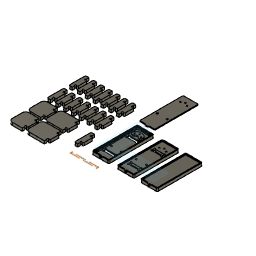
Basic Wood Geta with cavity v43 (Autodesk Fusion 360 design; units mm, degrees)
Autodesk Fusion 360 part; units mm, degrees
sketch "GetaDown" plane through (0, 0, 0) normal (0, 0, 1) x (1, 0, 0)
  line L0 (0, 0) -> (270, 0)
  line L1 (270, 0) -> (270, 100)
  line L2 (270, 100) -> (0, 100)
  line L3 (0, 100) -> (0, 0)
  line L4 (10, 90) -> (10, 10)
  line L5 (10, 10) -> (260, 10)
  line L6 (260, 10) -> (260, 90)
  line L7 (260, 90) -> (10, 90)
  dimension "d71" = 270
  dimension "d72" = 100
  constraint horizontal L0
  constraint vertical L1
  constraint horizontal L2
  constraint vertical L3
  constraint coincident L0.start L3.end
  measures "d71" distance of L0.start L0.end
  measures "d72" distance of L0.start L2.end
extrude "Extrude5" add sketch "GetaDown" along normal blind 5.6 contours L4 L5 L6 L7 makes body 1
extrude "Extrude12" add sketch "GetaDown" along normal blind 17.1 bodies 1
fillet "Fillet3" radius 6 4 edges at (0, 100, 8.55) (0, 0, 8.55) (270, 100, 8.55) (270, 0, 8.55) on bodies 1
fillet "Fillet7" radius 6 4 edges at (260, 90, 11.35) (260, 10, 11.35) (10, 90, 11.35) (10, 10, 11.35) on bodies 1
sketch "GetaUp" plane through (0, 0, 5.6) normal (0, 0, 1) x (-1, 0, 0)
  line L0 (0, 0) -> (-270, 0)
  line L1 (-270, 0) -> (-270, -100)
  line L2 (-270, -100) -> (0, -100)
  line L3 (0, -100) -> (0, 0)
  line L4 (-254, -90) -> (-16, -90)
  line L5 (-10, -84) -> (-10, -16)
  line L6 (-16, -10) -> (-254, -10)
  line L7 (-260, -16) -> (-260, -84)
  arc A0 (-10, -16) -> (-16, -10) centre (-16, -16) ccw
  arc A1 (-254, -10) -> (-260, -16) centre (-254, -16) ccw
  arc A2 (-260, -84) -> (-254, -90) centre (-254, -84) ccw
  arc A3 (-16, -90) -> (-10, -84) centre (-16, -84) ccw
  point P0 (-135, -90)
  point P1 (-135, -10)
  dimension "d17" = 270
  dimension "d18" = 100
  constraint horizontal L0
  constraint vertical L1
  constraint horizontal L2
  constraint vertical L3
  constraint midpoint L4 P0
  constraint midpoint L6 P1
  measures "d17" distance of L0.start L0.end
  measures "d18" distance of L0.start L2.end
extrude "Extrude7" add sketch "GetaUp" along normal blind 5 separate body contours L0 L1 L2 L3 | L4 L5 L6 L7 A0 A1 A2 A3 makes body 2
move_body "Move10" bodies 2 to x (1, 0, 0) y (0, 1, 0) z (0, 0, 1) at (0, 0, 17.1)
sketch "GetaBothPartHoles" plane through (0, 0, 5.6) normal (0, 0, 1) x (-1, 0, 0)
  circle A0 centre (-94.8, -80) radius 5
  circle A1 centre (-94.8, -20) radius 5
  circle A2 centre (-233.4, -50) radius 4
  circle A3 centre (-223.4, -70) radius 4
  circle A4 centre (-223.4, -30) radius 4
  line L0 (-254, -90) -> (-16, -90)
  line L1 (-10, -84) -> (-10, -16)
  line L2 (-16, -10) -> (-254, -10)
  line L3 (-260, -16) -> (-260, -84)
  arc A5 (-10, -16) -> (-16, -10) centre (-16, -16) ccw
  arc A6 (-254, -10) -> (-260, -16) centre (-254, -16) ccw
  arc A7 (-260, -84) -> (-254, -90) centre (-254, -84) ccw
  arc A8 (-16, -90) -> (-10, -84) centre (-16, -84) ccw
  line L4 (-10, -50) -> (-223.4, -50) construction
  line L5 (-223.4, -50) -> (-223.4, -70) construction
  line L6 (-223.4, -50) -> (-233.4, -50) construction
  line L7 (-223.4, -50) -> (-223.4, -30) construction
  dimension "d26" = 10
  dimension "d27" = 10
  dimension "d28" = 8
  dimension "d66" = 8
  dimension "d67" = 8
  dimension "d191" = 213.4
  dimension "d193" = 20
  dimension "d194" = 10
  dimension "d195" = 20
  constraint midpoint L1 L4.start
  constraint perpendicular L1 L4
  constraint vertical L5
  constraint horizontal L6
  constraint perpendicular L4 L7
  constraint coincident A2.centre L6.end
  constraint coincident A3.centre L5.end
  constraint coincident A4.centre L7.end
  measures "d26" diameter of A0
  measures "d27" diameter of A1
  measures "d28" diameter of A2
  measures "d66" diameter of A3
  measures "d67" diameter of A4
  measures "d191" distance of L4.start L4.end
  measures "d193" distance of L4.end A3.centre
  measures "d194" distance of L4.end A2.centre
  measures "d195" distance of L4.end A4.centre
extrude "Extrude9" cut sketch "GetaBothPartHoles" along normal mid plane 68.4 contours A0 | A1 | A2 | A3 | A4 bodies 1 2
sketch "GetaPillarShape" plane through (0, 0, 0) normal (1, 0, 0) x (0, 1, 0)
  line L0 (100, 0) -> (100, -20)
  line L1 (100, -20) -> (0, -20)
  line L2 (0, -20) -> (0, 0)
  line L3 (20, 0) -> (20, 12.1)
  line L4 (20, 12.1) -> (80, 12.1)
  line L5 (80, 12.1) -> (80, 0)
  line L6 (50, 0) -> (50, 20) construction
  line L7 (20, 0) -> (0, 0)
  line L8 (80, 0) -> (100, 0)
  circle A0 centre (80, 0) radius 4.5
  circle A1 centre (20, 0) radius 4.5
  dimension "d34" = 60
  dimension "d69" = 20
  dimension "d70" = 12.1
  dimension "d203" = 9
  dimension "d204" = 9
  constraint vertical L0
  constraint horizontal L1
  constraint vertical L2
  constraint coincident L2.end L7.end
  constraint symmetric L3 L5 L6
  constraint equal L3 L5
  constraint perpendicular L2 L7
  constraint perpendicular L0 L8
  constraint coincident L5.end L8.start
  constraint coincident L3.start L7.start
  measures "d34" distance of L5.end L3.start
  measures "d69" distance of L2.end L1.end
  measures "d70" distance of L5.end L4.end
  measures "d203" diameter of A0
  measures "d204" diameter of A1
extrude "Extrude10" add sketch "GetaPillarShape" along normal blind 16.8 separate body contours L0 L1 L2 L3 L4 L5 L7 L8 A0 A1 makes body 3
fillet "Fillet4" radius 6 2 edges at (8.4, 100, -20) (8.4, 0, -20) on bodies 3
fillet "Fillet6" radius 6 2 edges at (8.4, 80, 12.1) (8.4, 20, 12.1) on bodies 3
copy_body "CopyPasteBodies3" bodies 3 makes body 4
move_body "Move8" bodies 2 to x (1, 0, 0) y (0, 1, 0) z (0, 0, 1) at (0, 0, 10)
move_body "Move11" bodies 2 to x (1, 0, 0) y (0, 1, 0) z (0, 0, 1) at (0, 0, -20.6)
sketch "GetaDownTopMergeZone" plane through (0, 0, 0) normal (0, 0, 1) x (1, 0, 0)
  line L0 (265, 95) -> (5, 95)
  line L1 (5, 5) -> (265, 5)
  line L2 (265, 5) -> (265, 95)
  line L3 (5, 60) -> (0, 60)
  line L4 (0, 40) -> (5, 40)
  line L5 (5, 5) -> (5, 40)
  line L6 (5, 60) -> (5, 95)
  line L7 (0, 40) -> (0, 60)
  line L8 (0.0023, 4.8497) -> (5, 5) construction
  line L9 (5, 5) -> (5, 0) construction
  dimension "d90" = 20
  dimension "d198" = 5
  dimension "d199" = 5
  dimension "d200" = 260
  dimension "d201" = 90
  constraint parallel L3 L4
  constraint perpendicular L1 L5
  constraint perpendicular L0 L6
  constraint perpendicular L4 L7
  constraint equal L5 L6
  constraint equal L0 L1
  constraint perpendicular L1 L2
  constraint perpendicular L0 L2
  constraint perpendicular L1 L9
  measures "d90" distance of L3.end L4.start
  measures "d198" distance of L1.start L9.end
  measures "d199" distance of L1.start L8.start
  measures "d200" distance of L1.start L1.end
  measures "d201" distance of L0.start L1.end
extrude "Extrude15" add sketch "GetaDownTopMergeZone" along normal blind 5 separate body makes body 5
move_body "Move12" bodies 5 to x (1, 0, 0) y (0, 1, 0) z (0, 0, 1) at (0, 0, 12.1)
fillet "Fillet8" radius 3 8 edges at (5, 5, 14.6) (5, 40, 14.6) (0, 40, 14.6) (0, 60, 14.6) (5, 95, 14.6) (5, 60, 14.6) (265, 95, 14.6) (265, 5, 14.6) on bodies 5
combine "Combine3" operation cut target body 1 tool bodies 5 keep tools
combine "Combine4" operation intersect target body 2 tool bodies 5 keep tools
move_body "Move13" bodies 2 to x (1, 0, 0) y (0, 1, 0) z (0, 0, 1) at (0, 0, 20)
sketch "GetaHolesForPillar" plane through (0, 0, 0) normal (0, 0, 1) x (1, 0, 0)
  line L0 (0, 0) -> (270, 0) construction
  line L1 (270, 0) -> (270, 100) construction
  line L2 (270, 100) -> (0, 100) construction
  line L3 (0, 100) -> (0, 0) construction
  line L4 (45.9, 80) -> (63, 80)
  line L5 (63, 80) -> (63, 20)
  line L6 (63, 20) -> (45.9, 20)
  line L7 (45.9, 20) -> (45.9, 80)
  line L8 (45.9, 50) -> (0, 50) construction
  line L9 (186.3, 80) -> (203.1, 80)
  line L10 (203.1, 80) -> (203.1, 20)
  line L11 (203.1, 20) -> (186.3, 20)
  line L12 (186.3, 20) -> (186.3, 80)
  line L13 (186.3, 50) -> (0, 50) construction
  circle A0 centre (45.9, 80) radius 4.5
  circle A1 centre (63, 80) radius 4.5
  circle A2 centre (63, 20) radius 4.5
  circle A3 centre (45.9, 20) radius 4.5
  circle A4 centre (186.3, 20) radius 4.5
  circle A5 centre (203.1, 20) radius 4.5
  circle A6 centre (203.1, 80) radius 4.5
  circle A7 centre (186.3, 80) radius 4.5
  point P0 (45.9, 75.5)
  point P1 (50.4, 80)
  point P2 (58.5, 80)
  point P3 (63, 75.5)
  point P4 (58.5, 20)
  point P5 (63, 24.5)
  point P6 (50.4, 20)
  point P7 (45.9, 24.5)
  point P8 (190.8, 20)
  point P9 (186.3, 24.5)
  point P10 (198.6, 20)
  point P11 (203.1, 24.5)
  point P12 (198.6, 80)
  point P13 (203.1, 75.5)
  point P14 (186.3, 75.5)
  point P15 (190.8, 80)
  dimension "d167" = 270
  dimension "d168" = 100
  dimension "d169" = 17.1
  dimension "d170" = 60
  dimension "d171" = 45.9
  dimension "d172" = 16.8
  dimension "d173" = 60
  dimension "d174" = 186.3
  dimension "d179" = 9
  constraint horizontal L0
  constraint vertical L1
  constraint horizontal L2
  constraint vertical L3
  constraint coincident L0.start L3.end
  constraint horizontal L4
  constraint vertical L5
  constraint horizontal L6
  constraint vertical L7
  constraint midpoint L7 L8.start
  constraint midpoint L3 L8.end
  constraint perpendicular L3 L8
  constraint horizontal L9
  constraint vertical L10
  constraint horizontal L11
  constraint vertical L12
  constraint coincident L12 L13.start
  constraint coincident L3 L8.end
  constraint perpendicular L3 L13
  constraint symmetric L9 L11 L13
  constraint coincident L4.start L7.end
  constraint coincident L4.end L5.start
  constraint coincident L5.end L6.start
  constraint coincident L6.end L7.start
  constraint coincident L11.end L12.start
  constraint coincident L10.end L11.start
  constraint coincident L9.end L10.start
  constraint coincident L9.start L12.end
  constraint coincident A0 P0
  constraint coincident L7 P0
  constraint coincident A0 P1
  constraint coincident L4 P1
  constraint coincident A1 P2
  constraint coincident L4 P2
  constraint coincident A1 P3
  constraint coincident L5 P3
  constraint coincident L6 P4
  constraint coincident A2 P4
  constraint coincident L5 P5
  constraint coincident A2 P5
  constraint coincident A3 P6
  constraint coincident L6 P6
  constraint coincident A3 P7
  constraint coincident L11 P8
  constraint coincident A4 P8
  constraint coincident L12 P9
  constraint coincident A4 P9
  constraint coincident L11 P10
  constraint coincident A5 P10
  constraint coincident A5 P11
  constraint coincident L10 P11
  constraint coincident A6 P12
  constraint coincident L9 P12
  constraint coincident L10 P13
  constraint coincident A6 P13
  constraint coincident A7 P14
  constraint coincident L12 P14
  constraint coincident L9 P15
  constraint coincident A7 P15
  constraint equal A0 A1
  constraint equal A0 A2
  constraint equal A0 A3
  constraint equal A0 A7
  constraint equal A4 A7
  constraint equal A5 A7
  constraint equal A6 A7
  measures "d167" distance of L0.start L0.end
  measures "d168" distance of L0.start L2.end
  measures "d169" distance of L4.start L4.end
  measures "d170" distance of L4.start L6.end
  measures "d171" distance of L8.start L8.end
  measures "d172" distance of L9.start L9.end
  measures "d173" distance of L9.start L11.end
  measures "d174" distance of L8.end L13.start
  measures "d179" diameter of A0
extrude "Extrude17" cut sketch "GetaHolesForPillar" along normal blind 13.55 and the other way blind 13.55 bodies 1
move_body "Move17" bodies 4 to x (1, 0, 0) y (0, 1, 0) z (0, 0, 1) at (204.3, 0, 0)
move_body "Move18" bodies 3 to x (1, 0, 0) y (0, 1, 0) z (0, 0, 1) at (63.9, 0, 0)
sketch "WIP_FingersSupport" plane through (0, 0, 5.6) normal (0, 0, 1) x (-1, 0, 0)
  circle A0 centre (-223.4, -70) radius 4
  circle A1 centre (-233.4, -50) radius 4
  circle A2 centre (-223.4, -30) radius 4
  arc A3 (-10, -16) -> (-16, -10) centre (-16, -16) ccw
  line L0 (-16, -10) -> (-254, -10)
  arc A4 (-254, -10) -> (-260, -16) centre (-254, -16) ccw
  line L1 (-260, -16) -> (-260, -84)
  arc A5 (-260, -84) -> (-254, -90) centre (-254, -84) ccw
  line L2 (-254, -90) -> (-16, -90)
  arc A6 (-16, -90) -> (-10, -84) centre (-16, -84) ccw
  line L3 (-10, -84) -> (-10, -16)
  line L4 (-10, -90) -> (-223.4, -90) construction
  line L5 (-223.4, -90) -> (-223.4, -10)
  line L6 (-250, -10) -> (-250, -90)
  line L7 (-223.4, -10) -> (-250, -10)
  line L8 (-223.4, -90) -> (-250, -90)
  dimension "d208" = 213.4
  dimension "d209" = 26.6
  constraint coincident L2 L4.end
  constraint parallel L2 L4
  constraint coincident L0 L6.start
  constraint coincident L0 L5.end
  constraint coincident L2 L6.end
  constraint perpendicular L2 L6
  constraint perpendicular L6 L7
  measures "d208" distance of L4.start L4.end
  measures "d209" distance of L4.end L6.end
sketch "Reinforcement" plane through (0, 0, 5.6) normal (0, 0, 1) x (-1, 0, 0)
  line L0 (-203.1, -75.5) -> (-203.1, -24.5)
  arc A0 (-198.6, -20) -> (-203.1, -24.5) centre (-203.1, -20) ccw
  line L1 (-198.6, -20) -> (-190.8, -20)
  arc A1 (-186.3, -24.5) -> (-190.8, -20) centre (-186.3, -20) ccw
  line L2 (-186.3, -24.5) -> (-186.3, -75.5)
  arc A2 (-190.8, -80) -> (-186.3, -75.5) centre (-186.3, -80) ccw
  line L3 (-190.8, -80) -> (-198.6, -80)
  arc A3 (-203.1, -75.5) -> (-198.6, -80) centre (-203.1, -80) ccw
  line L4 (-63, -75.5) -> (-63, -24.5)
  arc A4 (-58.5, -20) -> (-63, -24.5) centre (-63, -20) ccw
  line L5 (-58.5, -20) -> (-50.4, -20)
  arc A5 (-45.9, -24.5) -> (-50.4, -20) centre (-45.9, -20) ccw
  line L6 (-45.9, -24.5) -> (-45.9, -75.5)
  arc A6 (-50.4, -80) -> (-45.9, -75.5) centre (-45.9, -80) ccw
  line L7 (-50.4, -80) -> (-58.5, -80)
  arc A7 (-63, -75.5) -> (-58.5, -80) centre (-63, -80) ccw
  circle A8 centre (-223.4, -70) radius 4
  circle A9 centre (-233.4, -50) radius 4
  circle A10 centre (-94.8, -20) radius 5
  circle A11 centre (-223.4, -30) radius 4
  circle A12 centre (-94.8, -80) radius 5
  arc A13 (-10, -16) -> (-16, -10) centre (-16, -16) ccw
  line L8 (-16, -10) -> (-254, -10)
  arc A14 (-254, -10) -> (-260, -16) centre (-254, -16) ccw
  line L9 (-260, -16) -> (-260, -84)
  arc A15 (-260, -84) -> (-254, -90) centre (-254, -84) ccw
  line L10 (-254, -90) -> (-16, -90)
  arc A16 (-16, -90) -> (-10, -84) centre (-16, -84) ccw
  line L11 (-10, -84) -> (-10, -16)
  arc A17 (-230.9335, -19.9553) -> (-230.9335, -80.0447) centre (-208.4, -50) ccw
  arc A18 (-215.8665, -40.0447) -> (-230.9335, -19.9553) centre (-223.4, -30) ccw
  arc A19 (-215.8665, -40.0447) -> (-215.8665, -59.9553) centre (-208.4, -50) ccw
  arc A20 (-230.9335, -80.0447) -> (-215.8665, -59.9553) centre (-223.4, -70) ccw
  arc A21 (-223.4, -30) -> (-223.4, -70) centre (-208.4, -50) ccw construction
  constraint tangent A17 A18
  constraint tangent A18 A19
  constraint tangent A19 A20
  constraint tangent A17 A20
  constraint coincident A11.centre A18.centre
  constraint coincident A8.centre A20.centre
extrude "Extrude18" add sketch "Reinforcement" along normal blind 6.5 separate body contours A17 A18 A19 A20 makes body 6
sketch "PowerCableHole" plane through (0, 0, 12.1) normal (0, 0, 1) x (-1, 0, 0)
  arc A0 (-16, -90) -> (-10, -84) centre (-16, -84) ccw
  line L0 (-16, -90) -> (-254, -90)
  arc A1 (-260, -84) -> (-254, -90) centre (-254, -84) ccw
  line L1 (-260, -84) -> (-260, -16)
  arc A2 (-254, -10) -> (-260, -16) centre (-254, -16) ccw
  line L2 (-254, -10) -> (-16, -10)
  arc A3 (-10, -16) -> (-16, -10) centre (-16, -16) ccw
  line L3 (-10, -16) -> (-10, -84)
  arc A4 (-262, -5) -> (-265, -8) centre (-262, -8) ccw
  line L4 (-265, -8) -> (-265, -92)
  arc A5 (-265, -92) -> (-262, -95) centre (-262, -92) ccw
  line L5 (-262, -95) -> (-8, -95)
  arc A6 (-8, -95) -> (-5, -92) centre (-8, -92) ccw
  line L6 (-5, -92) -> (-5, -62.9161)
  arc A7 (-2.5, -59.958) -> (-5, -62.9161) centre (-2, -62.9161) ccw
  arc A8 (-2.5, -59.958) -> (0, -57) centre (-3, -57) ccw
  line L7 (0, -57) -> (0, -42.9161)
  arc A9 (0, -42.9161) -> (-2.5, -39.958) centre (-3, -42.9161) ccw
  arc A10 (-5, -37) -> (-2.5, -39.958) centre (-2, -37) ccw
  line L8 (-5, -37) -> (-5, -8)
  arc A11 (-5, -8) -> (-8, -5) centre (-8, -8) ccw
  line L9 (-8, -5) -> (-262, -5)
  line L10 (-10, -55) -> (0, -55)
  line L11 (0, -45) -> (-10, -45)
  point P0 (0, -49.958)
  point P1 (-10, -50)
  point P2 (0, -55)
  point P3 (0, -45)
  point P4 (-10, -55)
  point P5 (-10, -45)
  constraint midpoint L7 P0
  constraint midpoint L3 P1
  constraint coincident L7 P2
  constraint coincident L7 P3
  constraint coincident L3 P4
  constraint coincident L3 P5
  constraint coincident P4 L10.start
  constraint coincident P2 L10.end
  constraint perpendicular L7 L10
  constraint coincident P3 L11.start
  constraint coincident P5 L11.end
  constraint perpendicular L3 L11
extrude "Extrude19" cut sketch "PowerCableHole" against normal blind 6 contours L3 L7 L10 L11 bodies 1
sketch "LaserCutableTopLines" plane through (0, 0, 37.1) normal (0, 0, 1) x (-1, 0, 0)
  arc A0 (0, -42.9161) -> (-2.5, -39.958) centre (-3, -42.9161) ccw
  arc A1 (-5, -37) -> (-2.5, -39.958) centre (-2, -37) ccw
  line L0 (-5, -37) -> (-5, -8)
  arc A2 (-5, -8) -> (-8, -5) centre (-8, -8) ccw
  line L1 (-8, -5) -> (-262, -5)
  arc A3 (-262, -5) -> (-265, -8) centre (-262, -8) ccw
  line L2 (-265, -8) -> (-265, -92)
  arc A4 (-265, -92) -> (-262, -95) centre (-262, -92) ccw
  line L3 (-262, -95) -> (-8, -95)
  arc A5 (-8, -95) -> (-5, -92) centre (-8, -92) ccw
  line L4 (-5, -92) -> (-5, -62.9161)
  arc A6 (-2.5, -59.958) -> (-5, -62.9161) centre (-2, -62.9161) ccw
  arc A7 (-2.5, -59.958) -> (0, -57) centre (-3, -57) ccw
  line L5 (0, -57) -> (0, -42.9161)
  circle A8 centre (-94.8, -80) radius 5
  circle A9 centre (-223.4, -30) radius 4
  circle A10 centre (-94.8, -20) radius 5
  circle A11 centre (-233.4, -50) radius 4
  circle A12 centre (-223.4, -70) radius 4
combine "Combine6" operation add target body 1 tool bodies 6 keep tools
copy_body "CopyPasteBodies4" bodies 3 makes body 7
move_body "Move19" bodies 7 to x (0, 0, -1) y (0, 1, 0) z (1, 0, 0) at (66.4, 150, 66.4)
move_body "Move20" bodies 7 to x (1, 0, 0) y (0, 1, 0) z (0, 0, 1) at (-46.4, -62, 31.4)
move_body "Move21" bodies 7 to x (1, 0, 0) y (0, 1, 0) z (0, 0, 1) at (0, 30, 0)
move_body "Move22" bodies 1 to x (0, 1, 0) y (-1, 0, 0) z (0, 0, 1) at (0, 0, 0)
copy_body "CopyPasteBodies5" bodies 1 makes body 8
move_body "Move23" bodies 8 to x (1, 0, 0) y (0, 1, 0) z (0, 0, 1) at (150, 0, 0)
extrude "Extrude20" add 1 faces at (90.9389, 154.6039, 5.6) along direction (0, 0, 1) blind 6.5 on bodies 8 bodies 8
move_body "Move24" bodies 7 to x (1, 0, 0) y (0, 1, 0) z (0, 0, 1) at (10, 50, 0)
copy_body "CopyPasteBodies6" bodies 7 makes body 9
copy_body "CopyPasteBodies7" bodies 8 makes body 10
move_body "Move25" bodies 10 to x (1, 0, 0) y (0, 1, 0) z (0, 0, 1) at (140, 0, 0)
sketch "Sketch28" plane through (0, 0, 0) normal (0, 0, 1) x (1, 0, 0)
  line L0 (285, 262) -> (195, 262)
  line L1 (195, 262) -> (195, 8)
  line L2 (195, 8) -> (285, 8)
  line L3 (285, 8) -> (285, 262)
  point P0 (285, 262)
  point P1 (195, 8)
  constraint horizontal L0
  constraint vertical L1
  constraint horizontal L2
  constraint vertical L3
  constraint coincident P1 L1.end
  constraint coincident P0 L0.start
extrude "Extrude21" add sketch "Sketch28" along normal blind 12.1 separate body makes body 11
combine "Combine7" operation add target body 10 tool bodies 11
move_body "Move27" bodies 7 to x (1, 0, 0) y (0, 1, 0) z (0, 0, 1) at (-10, -174, -17.1)
move_body "Move29" bodies 9 to x (1, 0, 0) y (0, 1, 0) z (0, 0, 1) at (-16, -168, -17.1)
move_body "Move30" bodies 9 to x (1, 0, 0) y (0, 1, 0) z (0, 0, 1) at (-400, 0, 0)
copy_body "CopyPasteBodies8" bodies 9 makes body 12
move_body "Move26" bodies 12 to x (1, 0, 0) y (0, 1, 0) z (0, 0, 1) at (-104.6061, 141.1196, 0)
pattern_linear "R-Pattern1" count 7 spacing 46.6667 along (1, 0, 0) count 2 spacing 130 along (0, 1, 0) of bodies 12 makes body 13 at (-458.5957, 200.4125, 16.8) makes body 14 at (-411.929, 200.4125, 16.8) makes body 15 at (-365.2624, 200.4125, 16.8) makes body 16 at (-318.5957, 200.4125, 16.8) makes body 17 at (-505.2624, 330.4125, 16.8) makes body 18 at (-458.5957, 330.4125, 16.8) makes body 19 at (-411.929, 330.4125, 16.8) makes body 20 at (-365.2624, 330.4125, 16.8) makes body 21 at (-318.5957, 330.4125, 16.8) makes body 22 at (-271.929, 200.4125, 16.8) makes body 23 at (-225.2624, 200.4125, 16.8) makes body 24 at (-271.929, 330.4125, 16.8) makes body 25 at (-225.2624, 330.4125, 16.8)
move_body "Move28" bodies 7 to x (1, 0, 0) y (0, 1, 0) z (0, 0, 1) at (-200, 0, 0)
sketch "MiLongPillar" plane through (0, 0, 0) normal (0, 0, -1) x (1, 0, 0)
  arc A0 (-373.9, -26) -> (-379.9, -20) centre (-379.9, -26) ccw
  line L0 (-379.9, -20) -> (-381.5, -20)
  arc A1 (-386, -15.5) -> (-381.5, -20) centre (-386, -20) ccw
  line L1 (-386, -15.5) -> (-386, 0)
  line L2 (-386, 0) -> (-400, 0)
  arc A2 (-400, 0) -> (-406, -6) centre (-400, -6) ccw
  line L3 (-400, -100) -> (-386, -100)
  line L4 (-386, -100) -> (-386, -84.5)
  arc A3 (-381.5, -80) -> (-386, -84.5) centre (-386, -80) ccw
  line L5 (-381.5, -80) -> (-379.9, -80)
  arc A4 (-379.9, -80) -> (-373.9, -74) centre (-379.9, -74) ccw
  line L6 (-373.9, -74) -> (-373.9, -26)
  line L7 (-386, -100) -> (-386, -84.5)
  line L8 (-386, -100) -> (-446, -100)
  line L9 (-386, -15.5) -> (-386, 0)
  line L10 (-386, 0) -> (-446, 0)
  line L11 (-466, -20) -> (-466, -80)
  line L12 (-373.9, -26) -> (-373.9, -74)
  arc A5 (-466, -80) -> (-446, -100) centre (-446, -80) ccw
  arc A6 (-446, 0) -> (-466, -20) centre (-446, -20) ccw
  point P0 (-466, -100)
  point P1 (-466, 0)
  dimension "d241" = 80
  dimension "d242" = 80
  dimension "d243" = 20
  constraint coincident L3.end L4.start
  constraint coincident L4.end A3.end
  constraint perpendicular L4 L8
  constraint coincident A1.start L1.start
  constraint coincident L1.end L2.start
  constraint perpendicular L1 L10
  constraint coincident A0.start L6.end
  constraint coincident A4.end L6.start
  constraint coincident P0 L11
  constraint coincident P0 L8
  constraint tangent L11 A5
  constraint tangent L8 A5
  constraint coincident P1 L10
  constraint coincident P1 L11
  constraint tangent L10 A6
  constraint tangent L11 A6
  constraint equal A5 A6
  measures "d241" distance of L3.end P0
  measures "d242" distance of L1.end P1
  measures "d243" radius of A5
extrude "Extrude22" add sketch "MiLongPillar" along normal blind 16.8 separate body makes body 26
sketch "LongPillar" plane through (0, 0, 0) normal (0, 0, 1) x (-1, 0, 0)
  line L0 (386, 0) -> (386, -15.5)
  arc A0 (381.5, -20) -> (386, -15.5) centre (386, -20) ccw
  line L1 (381.5, -20) -> (379.9, -20)
  arc A1 (379.9, -20) -> (373.9, -26) centre (379.9, -26) ccw
  line L2 (373.9, -26) -> (373.9, -74)
  arc A2 (373.9, -74) -> (379.9, -80) centre (379.9, -74) ccw
  line L3 (379.9, -80) -> (381.5, -80)
  arc A3 (386, -84.5) -> (381.5, -80) centre (386, -80) ccw
  line L4 (386, -84.5) -> (386, -100)
  line L5 (386, -100) -> (446, -100)
  arc A4 (446, -100) -> (466, -80) centre (446, -80) ccw
  line L6 (466, -80) -> (466, -20)
  arc A5 (466, -20) -> (446, 0) centre (446, -20) ccw
  line L7 (446, 0) -> (386, 0)
  line L8 (100, -264) -> (100, -6)
  line L9 (446, -100) -> (476, -100)
  line L10 (446, 0) -> (476, 0)
  line L11 (496, -20) -> (496, -80)
  arc A6 (476, -100) -> (496, -80) centre (476, -80) ccw
  arc A7 (496, -20) -> (476, 0) centre (476, -20) ccw
  point P0 (496, -100)
  point P1 (496, 0)
  dimension "d246" = 50
  dimension "d247" = 50
  dimension "d248" = 20
  dimension "d249" = 20
  constraint coincident L5.end A4.start
  constraint perpendicular L8 L9
  constraint coincident A5.end L7.start
  constraint parallel L7 L10
  constraint coincident P0 L9
  constraint coincident P0 L11
  constraint tangent L9 A6
  constraint tangent L11 A6
  constraint coincident P1 L10
  constraint coincident P1 L11
  constraint tangent L10 A7
  constraint tangent L11 A7
  measures "d246" distance of L5.end P0
  measures "d247" distance of A5.end P1
  measures "d248" radius of A6
  measures "d249" radius of A7
extrude "Extrude23" add sketch "LongPillar" along normal blind 16.8 separate body makes body 27
move_body "Move31" bodies 26 to x (1, 0, 0) y (0, 1, 0) z (0, 0, 1) at (-190, 0, 0)
move_body "Move32" bodies 26 to x (1, 0, 0) y (0, 1, 0) z (0, 0, 1) at (67.9, 0, 16.8)
move_body "Move33" bodies 26 to x (1, 0, 0) y (0, 1, 0) z (0, 0, 1) at (-10, 0, 0)
copy_body "CopyPasteBodies9" bodies 26 27 makes body 28 makes body 29
move_body "Move34" bodies 28 29 to x (1, 0, 0) y (0, 1, 0) z (0, 0, 1) at (0, 110, 0)
move_body "Move35" bodies 2 to x (0, 1, 0) y (-1, 0, 0) z (0, 0, 1) at (0, 0, 0)
sketch "LaserCutableTopLines 90 rot" plane through (0, 0, 37.1) normal (0, 0, 1) x (-1, 0, 0)
  arc A0 (42.9161, 0) -> (39.958, -2.5) centre (42.9161, -3) ccw
  arc A1 (37, -5) -> (39.958, -2.5) centre (37, -2) ccw
  line L0 (37, -5) -> (8, -5)
  arc A2 (8, -5) -> (5, -8) centre (8, -8) ccw
  line L1 (5, -8) -> (5, -262)
  arc A3 (5, -262) -> (8, -265) centre (8, -262) ccw
  line L2 (8, -265) -> (92, -265)
  arc A4 (92, -265) -> (95, -262) centre (92, -262) ccw
  line L3 (95, -262) -> (95, -8)
  arc A5 (95, -8) -> (92, -5) centre (92, -8) ccw
  line L4 (92, -5) -> (62.9161, -5)
  arc A6 (59.958, -2.5) -> (62.9161, -5) centre (62.9161, -2) ccw
  arc A7 (59.958, -2.5) -> (57, 0) centre (57, -3) ccw
  line L5 (57, 0) -> (42.9161, 0)
  circle A8 centre (80, -94.8) radius 5
  circle A9 centre (30, -223.4) radius 4
  circle A10 centre (20, -94.8) radius 5
  circle A11 centre (50, -233.4) radius 4
  circle A12 centre (70, -223.4) radius 4
sketch "Sketch32" plane through (0, 0, 0) normal (0, 0, 1) x (1, 0, 0)
  line L0 (-170.9186, -58.3177) -> (-14.527, -58.3177) construction
  line L1 (-14.527, -58.3177) -> (-14.527, -48.3177) construction
  line L2 (-14.527, -48.3177) -> (-170.9186, -48.3177) construction
  line L3 (-170.9186, -48.3177) -> (-170.9186, -58.3177) construction
  constraint perpendicular L0 L1
  constraint parallel L0 L2
  constraint parallel L1 L3
move_body "Move36" bodies 27 29 28 26 to x (1, 0, 0) y (0, 1, 0) z (0, 0, 1) at (90, -90, 0)
move_body "Move37" bodies 2 to x (1, 0, 0) y (0, 1, 0) z (0, 0, 1) at (0, 275, 0)
hidden bodies 3 4 5 6 9
equation "d15 = DownPartHeight - CavityHeightInShoe"
equation "d17 = ShoeLenght"
equation "d18 = ShoeWidth"
equation "d21 = TopPartHeight"
equation "d26 = HoleBackShoes"
equation "d27 = HoleBackShoes"
equation "d28 = HoleFrontShoes"
equation "d31 = DownPartHeight * 2"
equation "d34 = PillarHoleLenght"
equation "d36 = WoodPillartHiehgt"
equation "JoinTeethLenght = 10 mm"
equation "StringHoleSize = 8 mm"
equation "JoinTeethHeight = 3 mm"
equation "HoleFrontShoes = 8 mm"
equation "HoleBackShoes = 10 mm"
equation "ShoeLenght = 270 mm"
equation "ShoeWidth = 100 mm"
equation "TopPartHeight = 5 mm"
equation "DownPartHeight = 17.1 mm"
equation "BorderLength = 10 mm"
equation "CavityHeightInShoe = 11.5 mm"
equation "d64 = DownPartHeight"
equation "d66 = HoleFrontShoes"
equation "d67 = HoleFrontShoes"
equation "PillarExternalHeight = 20 mm"
equation "d69 = PillarExternalHeight"
equation "d70 = DownPartHeight - TopPartHeight"
equation "d71 = ShoeLenght"
equation "d72 = ShoeWidth"
equation "d73 = -BorderLength"
equation "d91 = TopPartHeight"
equation "d95 = DownPartHeight - TopPartHeight"
equation "DefaultFillet = 6 mm"
equation "SmallFillet = 6 mm"
equation "d103 = DefaultFillet"
equation "d104 = DefaultFillet"
equation "d106 = SmallFillet"
equation "dbToolDia = SmallFillet"
equation "dbOffset = 0 mm" comment "Do NOT change formula"
equation "dbRadius = ( dbToolDia + dbOffset ) / 2" comment "Do NOT change formula"
equation "dbMinPercent = 10"
equation "dbHoleOffset = dbRadius / sqrt(2)" comment "Do NOT change formula"
equation "d152 = DefaultFillet"
equation "PillarHoleLenght = ShoeWidth * 0.6"
equation "PillardHoleWidth = DownPartHeight"
equation "PourcentStartPillarBack = ShoeLenght * 0.17"
equation "PourcentStartPillarFront = ShoeLenght * 0.69"
equation "d167 = ShoeLenght"
equation "d168 = ShoeWidth"
equation "d169 = DownPartHeight"
equation "d170 = PillarHoleLenght"
equation "d171 = PourcentStartPillarBack"
equation "d172 = WoodPillartHiehgt"
equation "d173 = PillarHoleLenght"
equation "d174 = PourcentStartPillarFront"
equation "d177 = 5 mm + DownPartHeight / 2"
equation "d179 = SmallFillet * 1.5"
equation "d191 = PourcentStartPillarFront + DownPartHeight + 10 mm"
equation "HoleForwardDistance = 20 mm"
equation "d193 = HoleForwardDistance"
equation "d194 = HoleForwardDistance / 2"
equation "d195 = HoleForwardDistance"
equation "d196 = 5 mm + DownPartHeight / 2"
equation "d198 = BorderLength / 2"
equation "d199 = BorderLength / 2"
equation "d200 = ShoeLenght - 2 * BorderLength / 2"
equation "d201 = ShoeWidth - 2 * BorderLength / 2"
equation "d202 = SmallFillet / 2"
equation "d203 = SmallFillet * 1.5"
equation "d204 = SmallFillet * 1.5"
equation "StartFingerZone = PourcentStartPillarFront + DownPartHeight + 10 mm"
equation "FingerForceLenght = ShoeLenght - StartFingerZone - BorderLength * 3"
equation "d208 = StartFingerZone"
equation "d209 = FingerForceLenght"
equation "d216 = CavityHeightInShoe - TopPartHeight"
equation "CableHoleSize = 6 mm"
equation "d220 = -CableHoleSize"
equation "d226 = CavityHeightInShoe - TopPartHeight"
equation "d228 = DownPartHeight - TopPartHeight"
equation "WoodPillartHiehgt = 16.8 mm"
equation "d244 = WoodPillartHiehgt"
equation "d250 = WoodPillartHiehgt"
named bodies: "GetaDown", "GetaTop", "PillarBack", "Pillard", "PillarForward", "DownTopPartMergeZone", "Reinforcement", "PillarBack Copy", "GetaDown full", "PillarBack Copy (1)", "GetaDown full (1)", "PillarBack Copy (1) (1)", "PillarBack Copy (1) (1) (1)", "PillarBack Copy (1) (1) (2)", "PillarBack Copy (1) (1) (3)", "PillarBack Copy (1) (1) (4)", "PillarBack Copy (1) (1) (5)", "PillarBack Copy (1) (1) (6)", "PillarBack Copy (1) (1) (7)", "PillarBack Copy (1) (1) (8)", "PillarBack Copy (1) (1) (9)", "PillarBack Copy (1) (1) (10)", "PillarBack Copy (1) (1) (11)", "PillarBack Copy (1) (1) (12)", "PillarBack Copy (1) (1) (13)", "MiLongPillar", "LongPillar", "MiLongPillar (1)", "LongPillar (1)"
